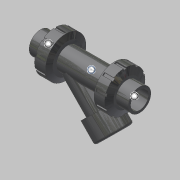
# Autodesk Inventor part: CHECK VALVE BALL GLUED DN25
Saved by Autodesk Inventor 2017 (Build 210142000, 142)
## iProperties
Created: 2016-04-26
Part Number: CHECK VALVE BALL GLUED DN25
Description: VRUIV VINK
Document SubType Name: Modeling
Manufacturer: SEKISUI
Mass: 197.859 g
Surface Area: 285.44 cm^2
Volume: 153.379 cm^3
Density: 1.29 g/cm^3
Material: U-PVC
Appearance: Smooth - Medium Gray
Catalog Web Link: http://www.pocketbrewery.com
Title: BALL VALVE PVC-U TRD DN15
Autodesk Inventor part; units mm, degrees
ref_plane "YZ Plane" through (0, 0, 0) normal (1, 0, 0) x (0, 1, 0)
ref_plane "XZ Plane" through (0, 0, 0) normal (0, 1, 0) x (-1, 0, 0)
ref_plane "XY Plane" through (0, 0, 0) normal (0, 0, 1) x (1, 0, 0)
sketch "Sketch_1" plane through (0, 0, 0) normal (1, 0, 0) x (0, 1, 0)
  line L0 (66, 0) -> (66, -24)
  line L1 (66, -24) -> (61.6324, -36)
  line L2 (61.6324, -36) -> (43.1265, -36)
  line L3 (43.1265, -36) -> (39.6, -26.3109)
  line L4 (39.6, -26.3109) -> (39.6, -16)
  line L5 (-39.6, -16) -> (-39.6, -26.3109)
  line L6 (-39.6, -26.3109) -> (-43.1265, -36)
  line L7 (-43.1265, -36) -> (-61.6324, -36)
  line L8 (-61.6324, -36) -> (-66, -24)
  line L9 (-66, -24) -> (-66, 0)
  line L10 (-66, 0) -> (66, 0)
  line L11 (-43.1265, -36) -> (0, -36) construction
  line L12 (0, -36) -> (0, -32) construction
  line L13 (-62.3603, -36) -> (-45.1265, -36)
  line L14 (-45.1265, -36) -> (-45.1265, -34)
  line L15 (-45.1265, -34) -> (-62.3603, -34)
  line L16 (-62.3603, -34) -> (-62.3603, -36)
  line L17 (45.1265, -36) -> (62.3603, -36)
  line L18 (62.3603, -36) -> (62.3603, -34)
  line L19 (62.3603, -34) -> (45.1265, -34)
  line L20 (45.1265, -34) -> (45.1265, -36)
  line L21 (-39.6, -16) -> (39.6, -16)
  point P0 (0, 0)
  point P1 (0, 0)
  point P2 (-52.3794, -36)
  point P3 (0, 0)
  dimension "dimZ" = 132
  dimension "dimE" = 72
  dimension "d22" = 36
  dimension "d23" = 12
  dimension "d24" = 20
  dimension "d27" = 26.4
  dimension "d28" = 26.4
  dimension "d40" = 4
  dimension "d52" = 20
  dimension "d53" = 2
  dimension "d54" = 2
  dimension "d55" = 2
  dimension "d73" = 32
  dimension "d74" = 12
  constraints: 44 end point, 6 parallel, 5 equal length, 5 horizontal, 5 perpendicular, 4 point on line, 3 collinear, 2 coincident, 2 midpoint
  measures "dimZ" distance of L9.end L0.start
  measures "dimE" diameter of L2 L10
  measures "d22" distance from line of L0.start L2
  measures "d23" vertical distance of L1.start L1.end
  measures "d24" angle of L0 L1
  measures "d27" distance between parallel lines of L9 L5
  measures "d28" distance between parallel lines of L0 L4
  measures "d40" distance of L11.end L12.end
  measures "d52" angle of L5 L6
  measures "d53" distance of L15.end L13.start
  measures "d54" distance from line of L6.end L14
  measures "d55" distance from line of L2.end L20
  measures "d73" diameter of L21 L10
  measures "d74" distance from line of L8.end L7
revolve "Revolution1" add sketch "Sketch_1" angle 360 about axis through (0, -66, 0) along (0, 1, 0) contours L0 L1 L19 L20 L2 L3 L4 L21 L5 L6 L7 L14 L15 L8 L9 L10 | L1 L2 L20 L19 | L15 L14 L7 L8 | L8 L13 L16
sketch "Sketch_7" plane through (0, 0, 0) normal (1, 0, 0) x (0, 1, 0)
  line L0 (-88, 20) -> (88, 20)
  line L1 (48.5126, 0) -> (-48.5126, 0)
  line L2 (-88, 20) -> (-88, 16)
  line L3 (-88, 16) -> (88, 16)
  line L4 (88, 16) -> (88, 20)
  line L5 (0, 0) -> (0, 20)
  point P0 (0, 16)
  dimension "dimH" = 176
  dimension "dimD" = 32
  dimension "dimD2" = 40
  constraints: 12 end point, 3 midpoint, 2 coincident, 2 perpendicular, 1 horizontal, 1 parallel, 1 point on line, 1 vertical
  measures "dimH" distance of L2.end L3.end
  measures "dimD" diameter of L3 L1
  measures "dimD2" diameter of L0 L1
revolve "Revolution3" add sketch "Sketch_7" angle 360 about axis through (0, 48.5126, 0) along (0, -1, 0)
extrude "Extrusion8" cut sketch "Sketch_1" along normal mid plane 4.8 contours L18 L17 L1 | L1 L2 L20 L19 | L15 L14 L7 L8 | L8 L13 L16
pattern_circular "Circular Pattern1" count 10 over 360 about axis through (0, 44, 0) along (0, -1, 0) of "Extrusion8"
sketch "Sketch16" plane through (0, 0, 0) normal (1, 0, 0) x (0, 1, 0)
  line L0 (-118.8997, -20) -> (-39.6, -20)
  line L1 (-39.6, -20) -> (28.1973, -89.41)
  line L2 (28.1973, -89.41) -> (42.5047, -75.4351)
  line L3 (42.5047, -75.4351) -> (-25.2926, -6.0251)
  line L4 (-25.2926, -6.0251) -> (-39.6, -20)
  line L5 (-25.2926, -6.0251) -> (-10.9853, 7.9499) construction
  line L6 (-10.9853, 7.9499) -> (56.8121, -61.4601) construction
  line L7 (56.8121, -61.4601) -> (42.5047, -75.4351) construction
  line L8 (-23.0518, 33.5326) -> (-22.7787, 35.7663) construction
  line L9 (28.1973, -89.41) -> (22.4744, -95)
  line L10 (22.4744, -95) -> (-1.9818, -69.9621)
  line L11 (-1.9818, -69.9621) -> (3.7412, -64.3721)
  line L12 (56.8121, -61.4601) -> (62.535, -55.8701) construction
  line L13 (62.535, -55.8701) -> (38.0789, -30.8322) construction
  line L14 (38.0789, -30.8322) -> (32.3559, -36.4222) construction
  line L15 (43.1265, -36) -> (43.1265, 36) projected
  line L16 (39.6, -20) -> (-39.6, -20) projected
  line L17 (0, -178.6) -> (0, 98.6) projected
  point P0 (0, 0)
  point P1 (0, 0)
  dimension "d75" = 40
  dimension "d77" = 8
  dimension "d78" = 35
  dimension "d79" = 3
  dimension "d80" = 95
  constraints: 30 end point, 10 perpendicular, 5 equal length, 3 point on line, 1 coincident, 1 collinear
  measures "d75" distance between parallel lines of L6 L1
  measures "d77" distance of L1.end L9.end
  measures "d78" distance of L9.end L10.end
  measures "d79" distance from line of L13 L8.end
  measures "d80" vertical distance of L9.end point (0, 0)
revolve "Revolution7" add sketch "Sketch16" angle 360 about axis through (0, 42.5047, -75.4351) along (0, -0.6987474, 0.7153685) contours L1 L17 L3 L2 | L1 L9 L10 L17 L11 | L1 L16 L3 L17 | L17 L10 L11 | L4 L3 L16
fillet "Fillet2" radius 3.2 1 edges at (0, 62.535, -55.8701)
equation "\"d23\" = 0.333333 * d22"
equation "\"d28\" = d27"
equation "\"d40\" = 0.333333 * d23"
equation "\"d47\" = 0.0666667 * dimE"
equation "\"oMe\" = dimE"
body "Solid1"
